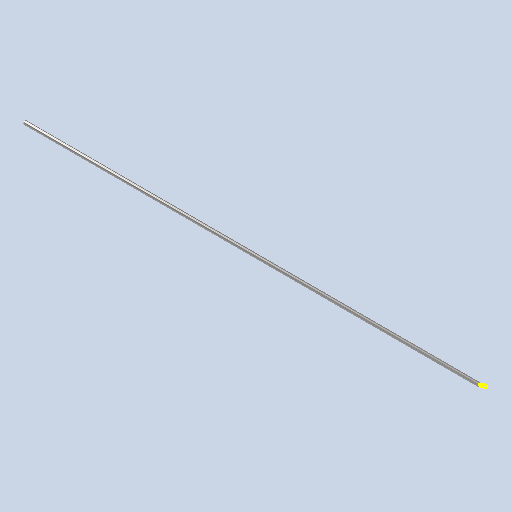
# Autodesk Inventor part: LeverArm
Saved by Autodesk Inventor 2023 (Build 270158000, 158)
## iProperties
Created: 2023-02-18
Part Number: LeverArm
Material: Stainless Steel
Document SubType Name: Modeling
Designer: phill
Density: 8 g/cm^3
Appearance: Semi-Polished
Author: phill
Autodesk Inventor part; units mm, degrees
ref_plane "YZ Plane" through (0, 0, 0) normal (1, 0, 0) x (0, 1, 0)
ref_plane "XZ Plane" through (0, 0, 0) normal (0, 1, 0) x (-1, 0, 0)
ref_plane "XY Plane" through (0, 0, 0) normal (0, 0, 1) x (1, 0, 0)
sketch "Sketch1" plane through (0, 0, 0) normal (0, 1, 0) x (-1, 0, 0)
  arc A0 (-4, 0) -> (0, 0) centre (-2, 0.1626) ccw projected
  line L0 (0, 0) -> (-4, 0) projected
sketch "Sketch2" plane through (0, 0, 0) normal (1, 0, 0) x (0, 1, 0)
  line L0 (0, 0) -> (-2.0066, 0)
  line L1 (-2.0066, 0) -> (-2.0066, -2.0066)
  line L2 (-2.0066, -2.0066) -> (0, -2.0066)
  line L3 (0, -2.0066) -> (0, 0)
  dimension "d0" = 2.0066
  dimension "d1" = 2.0066
  constraints: 8 end point, 2 parallel, 1 horizontal, 1 perpendicular
  measures "d0" distance of L1.end L2.end
  measures "d1" distance between parallel lines of L0 L2
extrude "Extrusion1" add sketch "Sketch2" against normal blind 250
fillet "Fillet1" radius 0.9906 4 edges at (-125, 0, 0) (-125, -2.0066, 0) (-125, 0, -2.0066) (-125, -2.0066, -2.0066)
body "Solid1"
